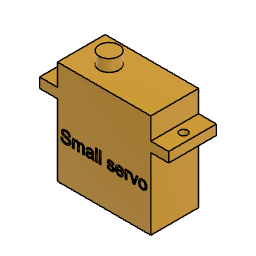
Small servo v1 (Autodesk Fusion 360 design; units mm, degrees)
Autodesk Fusion 360 part; units mm, degrees
sketch "Main body" plane through (0, 0, 0) normal (0, 0, 1) x (1, 0, 0)
  line L0 (0, 0) -> (23.5, 0)
  line L1 (23.5, 0) -> (23.5, 12)
  line L2 (23.5, 12) -> (0, 12)
  line L3 (0, 12) -> (0, 0)
  dimension "d1" = 23.5
  dimension "d2" = 12
  constraint horizontal L0
  constraint vertical L1
  constraint horizontal L2
  constraint vertical L3
  constraint coincident L0.start L3.end
  measures "d1" distance of L0.start L0.end
  measures "d2" distance of L0.start L2.end
extrude "Extrude1" add sketch "Main body" along normal blind 26
sketch "Horn base" plane through (0, 0, 26) normal (0, 0, 1) x (-1, 0, 0)
  line L0 (0, -12) -> (0, 0)
  line L1 (0, 0) -> (-23.5, 0)
  line L2 (-23.5, 0) -> (-23.5, -12)
  line L3 (-23.5, -12) -> (0, -12)
  circle A0 centre (-7, -6) radius 2.5
  dimension "d5" = 5
  dimension "d6" = 6
  dimension "d7" = 7
  measures "d5" diameter of A0
  measures "d6" distance of L3 A0.centre
  measures "d7" distance of L0 A0.centre
extrude "Extrude2" add sketch "Horn base" along normal blind 3 contours A0
sketch "Wing1" plane through (23.5, 0, 0) normal (1, 0, 0) x (0, 1, 0)
  line L0 (0, 0) -> (12, 0)
  line L1 (12, 0) -> (12, 26)
  line L2 (12, 26) -> (0, 26)
  line L3 (0, 26) -> (0, 0)
  line L4 (0, 20.5) -> (12, 20.5)
  line L5 (12, 20.5) -> (12, 18)
  line L6 (12, 18) -> (0, 18)
  line L7 (0, 18) -> (0, 20.5)
  dimension "d10" = 18
  dimension "d11" = 2.5
  constraint horizontal L4
  constraint vertical L5
  constraint horizontal L6
  constraint vertical L7
  constraint coincident L1 L5.end
  constraint coincident L3 L4.start
  measures "d10" distance of L0 L6
  measures "d11" distance of L4 L6
extrude "Wing1 (1)" add sketch "Wing1" along normal blind 4.5 contours L1 L3 L4 L5 L6 L7
sketch "Wing2" plane through (0, 0, 0) normal (-1, 0, 0) x (0, -1, 0)
  line L0 (-12, 0) -> (0, 0)
  line L1 (0, 0) -> (0, 26)
  line L2 (0, 26) -> (-12, 26)
  line L3 (-12, 26) -> (-12, 0)
  line L4 (-12, 20.5) -> (0, 20.5)
  line L5 (0, 20.5) -> (0, 18)
  line L6 (0, 18) -> (-12, 18)
  line L7 (-12, 18) -> (-12, 20.5)
  dimension "d14" = 18
  dimension "d15" = 2.5
  constraint horizontal L4
  constraint vertical L5
  constraint horizontal L6
  constraint vertical L7
  constraint coincident L1 L5.end
  constraint coincident L3 L4.start
  measures "d14" distance of L0 L6
  measures "d15" distance of L4 L6
extrude "Wing2 (1)" add sketch "Wing2" along normal blind 4.5 contours L1 L3 L4 L5 L6 L7
sketch "Holes" plane through (0, 0, 20.5) normal (0, 0, 1) x (-1, 0, 0)
  line L0 (-23.5, -12) -> (-23.5, 0)
  line L1 (-23.5, 0) -> (-28, 0)
  line L2 (-28, 0) -> (-28, -12)
  line L3 (-28, -12) -> (-23.5, -12)
  circle A0 centre (-25.75, -6) radius 1
  circle A1 centre (2.25, -6) radius 1
  line L4 (-11.75, -21) -> (-11.75, 10) construction
  line L5 (0, 0) -> (4.5, 0) construction
  dimension "d18" = 2
  dimension "d19" = 6
  dimension "d20" = 2
  dimension "d21" = 28
  dimension "d22" = 11.75
  dimension "d23" = 14
  dimension "d24" = 6
  constraint vertical L4
  measures "d18" diameter of A0
  measures "d19" distance of L1 A0.centre
  measures "d20" diameter of A1
  measures "d21" horizontal distance of A0.centre A1.centre
  measures "d22" distance of L0 L4
  measures "d23" distance of A0.centre L4
  measures "d24" distance of A1.centre L5
hole "Hole1" at (25.75, 6, 20.5) at (-2.25, 6, 20.5) direction (0, 0, -1) diameter 2 depth 2.5 tip angle 118
sketch "Text" plane through (0, 0, 0) normal (0, -1, 0) x (1, 0, 0)
  line L0 (0, 0) -> (23.5, 0)
  line L1 (23.5, 0) -> (23.5, 18)
  line L2 (23.5, 18) -> (28, 18)
  line L3 (28, 18) -> (28, 20.5)
  line L4 (28, 20.5) -> (23.5, 20.5)
  line L5 (23.5, 20.5) -> (23.5, 26)
  line L6 (23.5, 26) -> (0, 26)
  line L7 (0, 26) -> (0, 20.5)
  line L8 (0, 20.5) -> (-4.5, 20.5)
  line L9 (-4.5, 20.5) -> (-4.5, 18)
  line L10 (-4.5, 18) -> (0, 18)
  line L11 (0, 18) -> (0, 0)
  line L12 (0.8854, 7.9821) -> (33.8378, 7.6579) construction
  line L13 (33.8378, 7.6579) -> (33.8788, 11.8265) construction
  line L14 (33.8788, 11.8265) -> (0.9264, 12.1507) construction
  line L15 (0.9264, 12.1507) -> (0.8854, 7.9821) construction
  dimension "d28" = 3
  text T0 "Small servo" font "Arial" height 3 align left top in box 32.954 x 4.1688 at (0.8854, 7.9821) x (0.999952, -0.009837) y (0.009837, 0.999952) spacing 1
extrude "Extrude5" cut sketch "Text" against normal blind 1 text T0
